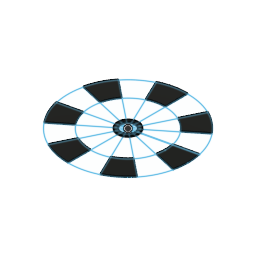
RPM_Pattern (Autodesk Fusion 360 design; units mm, degrees)
Autodesk Fusion 360 part; units mm, degrees
sketch "Sketch1" plane through (0, 0, 0) normal (0, 0, 1) x (1, 0, 0)
  circle A0 centre (0, 0) radius 7.5
  line L0 (-7.5, 0) -> (7.5, 0)
  line L1 (0, -7.5) -> (0, 7.5)
  circle A1 centre (0, 0) radius 39.75
  circle A2 centre (0, 0.0199) radius 63.75
  line L2 (11.7047, 2.6655) -> (62.1813, 14.0749)
  line L3 (0, 0) -> (62.1715, -14.0786)
  line L4 (0, 0) -> (49.7604, -39.8294)
  line L5 (0, 0.0199) -> (27.7367, -57.38)
  line L6 (0, 0) -> (-0.134, -63.73)
  line L7 (0, 0) -> (-27.5853, -57.4529)
  line L8 (0, 0) -> (-49.9274, -39.6199)
  line L9 (0, 0) -> (-62.1337, -14.2443)
  line L10 (0, 0.0199) -> (-62.1217, 14.3362)
  line L11 (0, 0) -> (-49.8925, 39.7037)
  line L12 (0, 0.0199) -> (-27.5393, 57.5146)
  line L13 (0, 0.0199) -> (-0.085, 63.7698)
  line L14 (0, 0.0199) -> (27.7807, 57.3984)
  line L15 (0, 0.0199) -> (49.7887, 39.8338)
  line L16 (11.7047, 2.6655) -> (0, 0)
  line L17 (0, 0) -> (62.1813, 14.0749)
  constraint coincident A0.centre A1.centre
  constraint coincident A0 L0.start
  constraint coincident A0 L0.end
  constraint horizontal L0
  constraint coincident A0 L1.start
  constraint coincident A0 L1.end
  constraint concentric A0 A1
  constraint coincident A2.centre L5.start
  constraint coincident A2 L2.end
  constraint coincident A2 L3.end
  constraint coincident A2 L4.end
  constraint coincident A2 L5.end
  constraint coincident A2 L6.end
  constraint coincident A2 L7.end
  constraint coincident A2 L8.end
  constraint coincident A2 L9.end
  constraint coincident A2 L10.end
  constraint coincident A2 L11.end
  constraint coincident A2 L12.end
  constraint coincident A2 L13.end
  constraint coincident A2 L14.end
  constraint coincident A2 L15.end
extrude "Extrude5" add sketch "Sketch1" along normal blind 1 contours A1 A2 L2 L3 L17 makes body 1
extrude "Extrude6" add sketch "Sketch1" along normal blind 1 separate body contours A1 A2 L14 L15 makes body 2
extrude "Extrude7" add sketch "Sketch1" along normal blind 1 separate body contours A1 A2 L12 L13 makes body 3
extrude "Extrude8" add sketch "Sketch1" along normal blind 1 separate body contours A1 A2 L10 L11 makes body 4
extrude "Extrude9" add sketch "Sketch1" along normal blind 1 separate body contours A1 A2 L8 L9 makes body 5
extrude "Extrude10" add sketch "Sketch1" along normal blind 1 separate body contours A1 A2 L6 L7 makes body 6
extrude "Extrude11" add sketch "Sketch1" along normal blind 1 separate body contours A1 A2 L4 L5 makes body 7
sketch "Sketch2" plane through (0, 0, 0) normal (0, 0, 1) x (1, 0, 0)
  circle A0 centre (0, 0) radius 7.5
  circle A1 centre (0, 0) radius 11
  dimension "d47" = 15
  dimension "d52" = 22
  constraint coincident A0.centre A1.centre
  measures "d47" diameter of A0
  measures "d52" diameter of A1
extrude "Extrude12" add sketch "Sketch2" along normal blind 1 separate body contours A0 makes body 8
extrude "Extrude13" cut 1 faces at (1.9158, 2.8099, 1) along direction (0, 0, -1) blind 1 on bodies 8 bodies 8
extrude "Extrude14" add sketch "Sketch2" along normal blind 1 bodies 8
